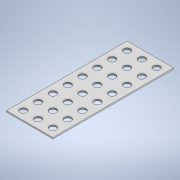
# Autodesk Inventor part: RackAdadpt
Saved by Autodesk Inventor 2020 (Build 240168000, 168)
## iProperties
Created: 2019-07-16
Part Number: RackAdadpt
Material: Generic
Document SubType Name: Modeling
Designer: eugen
Density: 1 g/cm^3
Appearance: Default
Author: eugen
Autodesk Inventor part; units mm, degrees
ref_plane "YZ Plane" through (0, 0, 0) normal (1, 0, 0) x (0, 1, 0)
ref_plane "XZ Plane" through (0, 0, 0) normal (0, 1, 0) x (-1, 0, 0)
ref_plane "XY Plane" through (0, 0, 0) normal (0, 0, 1) x (1, 0, 0)
sketch "Sketch1" plane through (0, 0, 0) normal (0, 1, 0) x (-1, 0, 0)
  line L0 (0, 0) -> (110.5662, 0)
  line L1 (110.5662, 0) -> (110.5662, -286.8422)
  line L2 (110.5662, -286.8422) -> (0, -286.8422)
  line L3 (0, -286.8422) -> (0, 0)
  circle A0 centre (90.5383, -20.0279) radius 8.128
  circle A1 centre (90.5383, -55.2831) radius 8.128
  circle A2 centre (90.5383, -90.5383) radius 8.128
  circle A3 centre (90.5383, -125.7935) radius 8.128
  circle A4 centre (90.5383, -161.0487) radius 8.128
  circle A5 centre (90.5383, -196.3039) radius 8.128
  circle A6 centre (90.5383, -231.5591) radius 8.128
  circle A7 centre (90.5383, -266.8143) radius 8.128
  circle A8 centre (55.2831, -20.0279) radius 8.128
  circle A9 centre (55.2831, -55.2831) radius 8.128
  circle A10 centre (55.2831, -90.5383) radius 8.128
  circle A11 centre (55.2831, -125.7935) radius 8.128
  circle A12 centre (55.2831, -161.0487) radius 8.128
  circle A13 centre (55.2831, -196.3039) radius 8.128
  circle A14 centre (55.2831, -231.5591) radius 8.128
  circle A15 centre (55.2831, -266.8143) radius 8.128
  circle A16 centre (20.0279, -20.0279) radius 8.128
  circle A17 centre (20.0279, -55.2831) radius 8.128
  circle A18 centre (20.0279, -90.5383) radius 8.128
  circle A19 centre (20.0279, -125.7935) radius 8.128
  circle A20 centre (20.0279, -161.0487) radius 8.128
  circle A21 centre (20.0279, -196.3039) radius 8.128
  circle A22 centre (20.0279, -231.5591) radius 8.128
  circle A23 centre (20.0279, -266.8143) radius 8.128
  dimension "d0" = 286.8422
  dimension "d1" = 110.5662
  dimension "d2" = 16.256
  dimension "d5" = 35.2552
  dimension "d8" = 35.2552
  dimension "d11" = 20.0279
  dimension "d12" = 20.0279
  constraints: 24 centre point, 8 end point, 2 horizontal, 2 parallel, 1 perpendicular, 1 vertical, 46 other
  measures "d0" distance of L0.end L1.end
  measures "d1" distance of L1.end L2.end
  measures "d2" diameter of A0
  measures "d5" distance of A0.centre A1.centre
  measures "d8" distance of A0.centre A8.centre
  measures "d11" horizontal distance of L0.end A0.centre
  measures "d12" distance from line of L0 A0.centre
extrude "Extrusion1" add sketch "Sketch1" along normal blind 3.175
equation "\"d12\" = d11"
body "Solid1"
